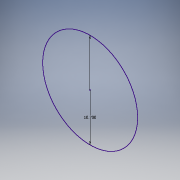
# Autodesk Inventor part: Ring Gear Outer
Saved by Autodesk Inventor 2016 (Build 200138000, 138)
## iProperties
Created: 2016-04-25
Part Number: Ring Gear Outer
Material: Generic
Document SubType Name: Modeling
Designer: rubenjm
Density: 1 g/cm^3
Appearance: Default
Author: rubenjm
Autodesk Inventor part; units mm, degrees
ref_plane "YZ Plane" through (0, 0, 0) normal (1, 0, 0) x (0, 1, 0)
ref_plane "XZ Plane" through (0, 0, 0) normal (0, 1, 0) x (-1, 0, 0)
ref_plane "XY Plane" through (0, 0, 0) normal (0, 0, 1) x (1, 0, 0)
sketch "Sketch1" plane through (0, 0, 0) normal (0, 0, 1) x (1, 0, 0)
  circle A0 centre (0, 0) radius 136.271
  circle A1 centre (0, 0) radius 190.5
  dimension "d0" = 272.542
  dimension "d1" = 381
  constraints: 2 centre point, 2 coincident
  measures "d0" diameter of A0
  measures "d1" diameter of A1
extrude "Extrusion1" add sketch "Sketch1" against normal blind 3.175
sketch "Sketch2" plane through (0, 0, 0) normal (0, 0, 1) x (1, 0, 0)
  circle A0 centre (0, 0) radius 157.48 construction
  circle A1 centre (-157.48, 0) radius 3.9687
  circle A2 centre (-78.74, -136.3817) radius 3.9687
  circle A3 centre (78.74, -136.3817) radius 3.9687
  circle A4 centre (157.48, 0) radius 3.9687
  circle A5 centre (78.74, 136.3817) radius 3.9687
  circle A6 centre (-78.74, 136.3817) radius 3.9687
  dimension "d6" = 314.96
  dimension "d7" = 7.9375
  dimension "d8" = 360
  constraints: 6 centre point, 1 coincident, 1 horizontal alignment, 15 other
  measures "d7" diameter of A1
extrude "Extrusion2" cut sketch "Sketch2" against normal through all
body "Solid1"
